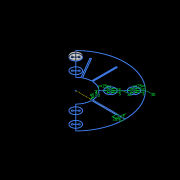
# Autodesk Inventor part: fin_alignment_rig_part3
Saved by Autodesk Inventor 2016 (Build 200138000, 138)
## iProperties
Created: 2024-02-20
Part Number: fin_alignment_rig_part3
Material: Generic
Document SubType Name: Modeling
Designer: kayla
Density: 1 g/cm^3
Appearance: Default
Author: kayla
Autodesk Inventor part; units mm, degrees
ref_plane "YZ Plane" through (0, 0, 0) normal (1, 0, 0) x (0, 1, 0)
ref_plane "XZ Plane" through (0, 0, 0) normal (0, 1, 0) x (-1, 0, 0)
ref_plane "XY Plane" through (0, 0, 0) normal (0, 0, 1) x (1, 0, 0)
sketch "Sketch1" plane through (0, 0, 0) normal (0, 0, 1) x (1, 0, 0)
  arc A0 (107.7631, -107.7631) -> (-107.7631, 107.7631) centre (0, 0) ccw
  line L0 (152.4, 0) -> (127, 0)
  line L1 (127, -1.66) -> (127, 1.66)
  line L2 (127, 1.66) -> (50.7729, 1.66)
  line L3 (50.7729, -1.66) -> (127, -1.66)
  line L4 (-64.9376, 109.1552) -> (-26.824, 43.1406)
  line L5 (-23.9488, 44.8006) -> (-62.0624, 110.8152)
  line L6 (-1.66, 127) -> (-1.66, 50.7729)
  line L7 (1.66, 50.7729) -> (1.66, 127)
  line L8 (1.66, 127) -> (-1.66, 127)
  line L9 (-62.0624, 110.8152) -> (-64.9376, 109.1552)
  line L10 (35.921, 35.921) -> (107.7631, 107.7631)
  line L11 (0, 0) -> (152.4, 0) construction
  line L12 (0, 0) -> (152.4, 0) construction
  line L13 (107.7631, -107.7631) -> (35.921, -35.921)
  line L14 (-35.921, 35.921) -> (-107.7631, 107.7631)
  arc A1 (-26.824, 43.1406) -> (-35.921, 35.921) centre (0, 0) ccw
  arc A2 (35.921, -35.921) -> (1.66, 50.7729) centre (0, 0) ccw
  arc A3 (-1.66, 50.7729) -> (-23.9488, 44.8006) centre (0, 0) ccw
  line L15 (35.921, 35.921) -> (53.5987, 53.5987)
  line L16 (107.7631, 107.7631) -> (90.0854, 90.0854)
  circle A4 centre (53.5987, 53.5987) radius 15
  line L17 (53.5987, 53.5987) -> (58.902, 48.2954)
  line L18 (53.5987, 53.5987) -> (48.2954, 58.902)
  circle A5 centre (48.2954, 58.902) radius 2.5
  circle A6 centre (58.902, 48.2954) radius 2.5
  circle A7 centre (90.0854, 90.0854) radius 15
  line L19 (90.0854, 90.0854) -> (95.3887, 84.7821)
  line L20 (90.0854, 90.0854) -> (84.7821, 95.3887)
  circle A8 centre (84.7821, 95.3887) radius 2.5
  circle A9 centre (95.3887, 84.7821) radius 2.5
  line L21 (-90.0854, 90.0854) -> (-84.7821, 95.3887)
  circle A10 centre (-84.7821, 95.3887) radius 2.5
  circle A11 centre (-90.0854, 90.0854) radius 15
  line L22 (-90.0854, 90.0854) -> (-95.3887, 84.7821)
  circle A12 centre (-95.3887, 84.7821) radius 2.5
  circle A13 centre (-58.902, 48.2954) radius 2.5
  circle A14 centre (-53.5987, 53.5987) radius 15
  line L23 (-53.5987, 53.5987) -> (-58.902, 48.2954)
  circle A15 centre (-48.2954, 58.902) radius 2.5
  line L24 (-53.5987, 53.5987) -> (-48.2954, 58.902)
  line L25 (90.0854, -90.0854) -> (84.7821, -95.3887)
  circle A16 centre (84.7821, -95.3887) radius 2.5
  circle A17 centre (90.0854, -90.0854) radius 15
  line L26 (90.0854, -90.0854) -> (95.3887, -84.7821)
  circle A18 centre (95.3887, -84.7821) radius 2.5
  circle A19 centre (58.902, -48.2954) radius 2.5
  circle A20 centre (53.5987, -53.5987) radius 15
  line L27 (53.5987, -53.5987) -> (58.902, -48.2954)
  circle A21 centre (48.2954, -58.902) radius 2.5
  line L28 (53.5987, -53.5987) -> (48.2954, -58.902)
  point P0 (50.8, 0)
  dimension "d2" = 25.4
  dimension "d3" = 3.32
  dimension "d10" = 45
  dimension "d12" = 25
  dimension "d13" = 25
  dimension "d14" = 30
  dimension "d15" = 7.5
  dimension "d16" = 7.5
  dimension "d17" = 5
  dimension "d18" = 5
  dimension "d19" = 30
  dimension "d20" = 7.5
  dimension "d21" = 7.5
  dimension "d22" = 5
  dimension "d23" = 5
  constraints: 58 end point, 22 centre point, 14 coincident, 14 point on circle, 5 horizontal, 2 point on line, 1 parallel, 1 perpendicular
  measures "d2" distance of L0.start L0.end
  measures "d3" distance of L1.end L1.start
  measures "d10" angle of L11 L10
  measures "d12" distance of L10.start L15.end
  measures "d13" distance of L10.end L16.end
  measures "d14" diameter of A4
  measures "d15" distance of L17.start L17.end
  measures "d16" distance of L17.start L18.end
  measures "d17" diameter of A5
  measures "d18" diameter of A6
  measures "d19" diameter of A7
  measures "d20" distance of L19.start L19.end
  measures "d21" distance of L19.start L20.end
  measures "d22" diameter of A8
  measures "d23" diameter of A9
extrude "Extrusion5" add sketch "Sketch1" along normal blind 3 contours A11 L14 | L14 A11
body "Solid2"
body "Solid3"
